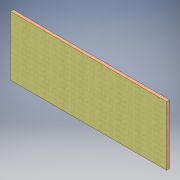
# Autodesk Inventor part: computerTop
Saved by Autodesk Inventor 2017 (Build 210142000, 142)
## iProperties
Created: 2018-09-10
Part Number: computerTop
Material: Wood (Birch)
Document SubType Name: Modeling
Designer: emmacarlisle
Density: 0.55 g/cm^3
Appearance: Birch - Natural Polished
Author: emmacarlisle
Autodesk Inventor part; units mm, degrees
ref_plane "YZ Plane" through (0, 0, 0) normal (1, 0, 0) x (0, 1, 0)
ref_plane "XZ Plane" through (0, 0, 0) normal (0, 1, 0) x (-1, 0, 0)
ref_plane "XY Plane" through (0, 0, 0) normal (0, 0, 1) x (1, 0, 0)
sketch "Sketch1" plane through (0, 0, 0) normal (0, 0, 1) x (1, 0, 0)
  line L0 (0, 0) -> (2100, 0)
  line L1 (2100, 0) -> (2100, 800)
  line L2 (2100, 800) -> (0, 800)
  line L3 (0, 800) -> (0, 0)
  dimension "d0" = 2100
  dimension "d1" = 800
  constraints: 8 end point, 2 parallel, 1 horizontal, 1 perpendicular
  measures "d0" distance of L1.end L2.end
  measures "d1" distance of L2.end L0.start
extrude "Extrusion1" add sketch "Sketch1" along normal blind 40
body "Solid1"
